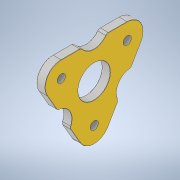
# Autodesk Inventor part: Torque_Triangle
Saved by Autodesk Inventor 2021 (Build 250183000, 183)
## iProperties
Created: 2020-10-13
Part Number: Torque_Triangle
Material: Generic
Document SubType Name: Modeling
Designer: PhotonUser
Density: 1 g/cm^3
Appearance: Default
Author: PhotonUser
Autodesk Inventor part; units mm, degrees
ref_plane "YZ Plane" through (0, 0, 0) normal (1, 0, 0) x (0, 1, 0)
ref_plane "XZ Plane" through (0, 0, 0) normal (0, 1, 0) x (-1, 0, 0)
ref_plane "XY Plane" through (0, 0, 0) normal (0, 0, 1) x (1, 0, 0)
sketch "Sketch1" plane through (0, 0, 0) normal (1, 0, 0) x (0, 1, 0)
  circle A0 centre (0, -62.2579) radius 15.875
  circle A1 centre (18.7452, -94.7256) radius 4.0043
  circle A2 centre (18.7452, -94.7256) radius 15.875
  circle A3 centre (-37.4904, -62.2579) radius 4.0043
  circle A4 centre (-37.4904, -62.2579) radius 15.875
  circle A5 centre (18.7452, -29.7903) radius 15.875
  circle A6 centre (18.7452, -29.7903) radius 4.0043
  circle A7 centre (18.7452, -94.7256) radius 4.0043
  circle A8 centre (18.7452, -94.7256) radius 15.875
  circle A9 centre (0, -62.2579) radius 15.875
  circle A10 centre (-37.4904, -62.2579) radius 4.0043
  circle A11 centre (-37.4904, -62.2579) radius 15.875
  circle A12 centre (18.7452, -29.7903) radius 4.0043
  circle A13 centre (18.7452, -29.7903) radius 15.875
  line L0 (34.6202, -29.7903) -> (34.6202, -94.7256)
  line L1 (10.8077, -108.4737) -> (-45.4279, -76.0061)
  line L2 (10.8077, -16.0421) -> (-45.4279, -48.5098)
  circle A14 centre (18.7452, -29.7903) radius 15.875
  circle A15 centre (-37.4904, -62.2579) radius 15.875
  circle A16 centre (18.7452, -94.7256) radius 15.875
  circle A17 centre (41.995, -62.2579) radius 14.4142
  circle A18 centre (-20.9975, -25.8892) radius 14.4142
  circle A19 centre (-20.9975, -98.6266) radius 14.4142
  point P0 (-28.0356, -86.0475)
  point P1 (-6.5846, -98.4323)
  point P2 (34.6202, -74.6426)
  point P3 (34.6202, -49.8732)
  point P4 (-6.5846, -26.0836)
  point P5 (-28.0356, -38.4683)
  point P6 (-45.4279, -48.5098)
  dimension "d28" = 360
  constraints: 20 centre point, 7 coincident, 7 concentric, 7 tangent, 6 end point, 6 point on circle, 7 other
extrude "Extrusion1" add sketch "Sketch1" along normal blind 8.255 contours A2 | A2 L1 A19 A4 L2 A18 A5 L0 A17 | A5 | A4
fillet "Fillet2" radius 3.175 6 edges at (4.1275, 34.6202, -49.8732) (4.1275, 34.6202, -74.6426) (4.1275, -6.5846, -26.0836) (4.1275, -28.0356, -38.4683) (4.1275, -6.5846, -98.4323) (4.1275, -28.0356, -86.0475)
chamfer "Chamfer3" distance 0.254 angle 45 38 edges at (8.255, 2.8431, -103.8753) (8.255, 26.6827, -108.4737) (8.255, 34.6202, -85.5288) (8.255, 34.2848, -74.9118) (8.255, 27.5808, -62.2579) (8.255, 34.2848, -49.604) (8.255, 34.6202, -38.987) (8.255, 26.6827, -16.0421) (8.255, 2.8431, -20.6405) (8.255, -6.1838, -26.2395) (8.255, -13.7904, -38.3722) (8.255, -28.101, -38.8933) (8.255, -37.4633, -43.9114) (8.255, -53.3654, -62.2579) (8.255, -37.4633, -80.6044) (8.255, -28.101, -85.6225) (8.255, -13.7904, -86.1436) (8.255, -6.1838, -98.2764) (0, 2.8431, -103.8753) (0, 26.6827, -108.4737) (0, 34.6202, -85.5288) (0, 34.2848, -74.9118) (0, 27.5808, -62.2579) (0, 34.2848, -49.604) (0, 34.6202, -38.987) (0, 26.6827, -16.0421) (0, 2.8431, -20.6405) (0, -6.1838, -26.2395) (0, -13.7904, -38.3722) (0, -28.101, -38.8933) (0, -37.4633, -43.9114) (0, -53.3654, -62.2579) (0, -37.4633, -80.6044) (0, -28.101, -85.6225) (0, -13.7904, -86.1436) (0, -6.1838, -98.2764) (0, -15.875, -62.2579) (8.255, -15.875, -62.2579)
body "Solid1"
